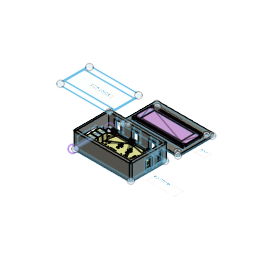
FurModularity case (Autodesk Fusion 360 design; units mm, degrees)
part number: 2026-01-23-19-48-48-350
Autodesk Fusion 360 part; units mm, degrees
sketch "Esboço1" plane through (0, 0, 0) normal (0, 1, 0) x (1, 0, 0)
  line L0 (-156.1961, 83) -> (-258.1961, 83)
  line L1 (-258.1961, 83) -> (-258.1961, 23)
  line L2 (-258.1961, 23) -> (-156.1961, 23)
  line L3 (-156.1961, 23) -> (-156.1961, 83)
  line L4 (-261.1961, 88) -> (-151.1961, 88)
  line L5 (-151.1961, 88) -> (-151.1961, 18)
  line L6 (-151.1961, 18) -> (-261.1961, 18)
  line L7 (-261.1961, 18) -> (-261.1961, 88)
  circle A0 centre (-258.6961, 20.5) radius 1.7
  circle A1 centre (-153.6961, 20.5) radius 1.7
  circle A2 centre (-153.6961, 85.5) radius 1.7
  circle A3 centre (-258.6961, 85.5) radius 1.7
  line L8 (-382.0556, 170.4962) -> (-284.0556, 170.4962)
  line L9 (-284.0556, 170.4962) -> (-284.0556, 110.4962)
  line L10 (-284.0556, 110.4962) -> (-382.0556, 110.4962)
  line L11 (-382.0556, 110.4962) -> (-382.0556, 170.4962)
  circle A4 centre (-379.5556, 167.9962) radius 1.25
  circle A5 centre (-379.5556, 112.9962) radius 1.25
  circle A6 centre (-286.5556, 112.9962) radius 1.25
  circle A7 centre (-286.5556, 167.9962) radius 1.25
  line L12 (-380.2556, 159.1962) -> (-285.8556, 159.1962)
  line L13 (-285.8556, 159.1962) -> (-285.8556, 121.7962)
  line L14 (-285.8556, 121.7962) -> (-380.2556, 121.7962)
  line L15 (-380.2556, 121.7962) -> (-380.2556, 159.1962)
  line L16 (-148.0106, 174.0206) -> (-148.0106, 104.0206)
  line L17 (-148.0106, 104.0206) -> (-258.0106, 104.0206)
  line L18 (-258.0106, 104.0206) -> (-258.0106, 174.0206)
  line L19 (-258.0106, 174.0206) -> (-148.0106, 174.0206)
  circle A8 centre (-255.5106, 171.5206) radius 1.5
  circle A9 centre (-150.5106, 171.5206) radius 1.5
  circle A10 centre (-255.5106, 106.5206) radius 1.5
  circle A11 centre (-150.5106, 106.5206) radius 1.5
  line L20 (-348.3038, 137.4104) -> (-309.3267, 137.4104) construction
  line L21 (-309.3267, 137.4104) -> (-309.3267, 143.3671) construction
  line L22 (-309.3267, 143.3671) -> (-348.3038, 143.3671) construction
  line L23 (-348.3038, 143.3671) -> (-348.3038, 137.4104) construction
  line L24 (-139.2514, 36.3126) -> (-87.0034, 36.3126) construction
  line L25 (-87.0034, 36.3126) -> (-87.0034, 53) construction
  line L26 (-87.0034, 53) -> (-139.2514, 53) construction
  line L27 (-139.2514, 53) -> (-139.2514, 36.3126) construction
  circle A12 centre (-249.5106, 111.5206) radius 1.25
  line L28 (-155.8106, 120.3206) -> (-250.2106, 120.3206)
  line L29 (-250.2106, 157.7206) -> (-155.8106, 157.7206)
  line L30 (-250.2106, 120.3206) -> (-250.2106, 157.7206)
  circle A13 centre (-156.5106, 166.5206) radius 1.25
  circle A14 centre (-249.5106, 166.5206) radius 1.25
  circle A15 centre (-156.5106, 111.5206) radius 1.25
  line L31 (-155.8106, 157.7206) -> (-155.8106, 120.3206)
  line L32 (-140, 128.1599) -> (-121.0217, 128.1599) construction
  line L33 (-121.0217, 128.1599) -> (-121.0217, 140) construction
  line L34 (-121.0217, 140) -> (-140, 140) construction
  line L35 (-140, 140) -> (-140, 128.1599) construction
  dimension "d17" = 60
  dimension "d18" = 102
  dimension "d19" = 110
  dimension "d20" = 70
  dimension "d22" = 5
  dimension "d25" = 3.4
  dimension "d27" = 2.5
  dimension "d28" = 2.5
  dimension "d29" = 3.4
  dimension "d30" = 2.5
  dimension "d31" = 2.5
  dimension "d32" = 3.4
  dimension "d33" = 3.4
  dimension "d34" = 2.5
  dimension "d35" = 2.5
  dimension "d36" = 2.5
  dimension "d37" = 2.5
  dimension "d54" = 60
  dimension "d55" = 98
  dimension "d60" = 2.5
  dimension "d61" = 2.5
  dimension "d62" = 2.5
  dimension "d63" = 2.5
  dimension "d64" = 2.5
  dimension "d65" = 2.5
  dimension "d66" = 2.5
  dimension "d67" = 2.5
  dimension "d68" = 2.5
  dimension "d69" = 2.5
  dimension "d70" = 2.5
  dimension "d71" = 2.5
  dimension "d73" = 94.4
  dimension "d74" = 37.4
  dimension "d75" = 1.8
  dimension "d76" = 11.3
  dimension "d77" = 70
  dimension "d78" = 110
  dimension "d79" = 3
  dimension "d80" = 3
  dimension "d82" = 3
  dimension "d83" = 2.5
  dimension "d85" = 2.5
  dimension "d86" = 2.5
  dimension "d87" = 2.5
  dimension "d88" = 3
  dimension "d89" = 2.5
  dimension "d90" = 2.5
  dimension "d91" = 2.5
  dimension "d92" = 2.5
  dimension "d93" = 5
  dimension "d94" = 0
  dimension "d95" = 5
  dimension "d105" = 2.5
  dimension "d108" = 2.5
  dimension "d111" = 2.5
  dimension "d114" = 2.5
  dimension "d117" = 94.4
  dimension "d118" = 37.4
  dimension "d121" = 93
  dimension "d122" = 55
  dimension "d124" = 93
  dimension "d125" = 8.8
  dimension "d126" = 8.8
  dimension "d127" = 0.7
  dimension "d129" = 7.5
  dimension "d132" = 5
  dimension "d135" = 8.5
  dimension "d173" = 5
  constraint horizontal L0
  constraint vertical L1
  constraint horizontal L2
  constraint vertical L3
  constraint horizontal L4
  constraint vertical L5
  constraint horizontal L6
  constraint vertical L7
  constraint horizontal L8
  constraint vertical L9
  constraint horizontal L10
  constraint vertical L11
  constraint horizontal L12
  constraint vertical L13
  constraint horizontal L14
  constraint vertical L15
  constraint vertical L16
  constraint horizontal L17
  constraint vertical L18
  constraint perpendicular L16 L19
  constraint horizontal L29
  constraint vertical L31
  constraint horizontal L28
  constraint vertical L30
  measures "d17" distance of L0.start L2.end
  measures "d18" distance of L0.start L0.end
  measures "d19" distance of L4.start L4.end
  measures "d20" distance of L4.start L6.end
  measures "d22" distance of L0 L4
  measures "d25" diameter of A0
  measures "d27" distance of L7 A0.centre
  measures "d28" distance of L6 A0.centre
  measures "d29" diameter of A1
  measures "d30" distance of L5 A1.centre
  measures "d31" distance of L6 A1.centre
  measures "d32" diameter of A3
  measures "d33" diameter of A2
  measures "d34" distance of L4 A2.centre
  measures "d35" distance of L5 A2.centre
  measures "d36" distance of L4 A3.centre
  measures "d37" distance of L7 A3.centre
  measures "d54" distance of L8.start L10.end
  measures "d55" distance of L8.start L8.end
  measures "d60" diameter of A4
  measures "d61" distance of L8 A4.centre
  measures "d62" distance of L11 A4.centre
  measures "d63" diameter of A5
  measures "d64" distance of L10 A5.centre
  measures "d65" distance of L11 A5.centre
  measures "d66" diameter of A6
  measures "d67" distance of L9 A6.centre
  measures "d68" distance of L10 A6.centre
  measures "d69" diameter of A7
  measures "d70" distance of L8 A7.centre
  measures "d71" distance of L9 A7.centre
  measures "d73" distance of L12.start L12.end
  measures "d74" distance of L12.start L14.end
  measures "d75" distance of L11 L15
  measures "d76" distance of L10 L14
  measures "d77" distance of L18.end L17.end
  measures "d78" distance of L18.end L16.start
  measures "d79" diameter of A8
  measures "d80" diameter of A9
  measures "d82" diameter of A10
  measures "d83" distance of L19 A8.centre
  measures "d85" distance of L18 A8.centre
  measures "d86" distance of L19 A9.centre
  measures "d87" distance of L16 A9.centre
  measures "d88" diameter of A11
  measures "d89" distance of L16 A11.centre
  measures "d90" distance of L17 A11.centre
  measures "d91" distance of L17 A10.centre
  measures "d92" distance of L18 A10.centre
  measures "d105" diameter of A14
  measures "d108" diameter of A12
  measures "d111" diameter of A15
  measures "d114" diameter of A13
  measures "d117" distance of L29.start L29.end
  measures "d118" distance of L29.start L28.end
  measures "d121" distance of A15.centre A12.centre
  measures "d122" distance of A14.centre A12.centre
  measures "d124" distance of A14.centre A13.centre
  measures "d125" distance of A14.centre L29
  measures "d126" distance of A15.centre L28
  measures "d127" distance of A14.centre L30
  measures "d129" distance of L19 A14.centre
  measures "d135" distance of L18 A14.centre
  measures "d173" distance of L3 L5
other "Recurso de malha base1"
other "Modificar1"
other "Modificar2"
other "Modificar3"
other "Modificar4"
other "Recurso de malha base2"
other "Modificar5"
other "Modificar6"
other "Modificar7"
other "Modificar8"
extrude "Extrusão18" add sketch "Esboço1" along normal blind 30 contours L4 L5 L6 L7 makes body 1
extrude "Extrusão19" add sketch "Esboço1" along normal blind 3 separate body contours L0 L1 L2 L3 | A0 | A1 | A2 | A3 makes body 2 at (-258.2357, 2, -87.1365) makes body 3 at (-153.6537, 2, -87.1995) makes body 4 at (-258.2357, 2, -22.1365) makes body 5 at (-190.1961, 0, -63) makes body 6 at (-153.6537, 2, -22.1995)
sketch "Esboço4" plane through (-261.1961, 0, 0) normal (-1, 0, 0) x (0, 0, 1)
  line L0 (-88, 0) -> (-18, 0)
  line L1 (-18, 0) -> (-18, 30)
  line L2 (-18, 30) -> (-88, 30)
  line L3 (-88, 30) -> (-88, 0)
  line L4 (-18, 0) -> (-88, 0)
  line L5 (-73.7635, 9.0114) -> (-62.7635, 9.0114)
  line L6 (-62.7635, 9.0114) -> (-62.7635, 2.0114)
  line L7 (-62.7635, 2.0114) -> (-73.7635, 2.0114)
  line L8 (-73.7635, 2.0114) -> (-73.7635, 9.0114)
  line L9 (-61.7, 16.0562) -> (-27.0978, 16.0562)
  line L10 (-27.0978, 16.0562) -> (-27.0978, 3.9829)
  line L11 (-27.0978, 3.9829) -> (-61.7, 3.9829)
  line L12 (-61.7, 3.9829) -> (-61.7, 16.0562)
  point P0 (-58.6316, 10.8)
  dimension "d184" = 7
  dimension "d185" = 11
  constraint horizontal L5
  constraint vertical L6
  constraint horizontal L7
  constraint vertical L8
  constraint horizontal L9
  constraint vertical L10
  constraint horizontal L11
  constraint vertical L12
  measures "d184" distance of L5 L7
  measures "d185" distance of L6 L8
extrude "Extrusão20" cut sketch "Esboço4" against normal blind 3 contours L5 L6 L7 L8 | L9 L10 L11 L12 bodies 1
extrude "Extrusão21" add sketch "Esboço1" along normal blind 3 separate body contours L16 L17 L18 L19 makes body 7
sketch "Esboço5" plane through (0, 0, -88) normal (0, 0, -1) x (-1, 0, 0)
  line L0 (151.1961, 0) -> (261.1961, 0)
  line L1 (261.1961, 0) -> (261.1961, 30)
  line L2 (261.1961, 30) -> (151.1961, 30)
  line L3 (151.1961, 30) -> (151.1961, 0)
  line L4 (170.1901, 3.9119) -> (182.6901, 3.9119)
  line L5 (182.6901, 3.9119) -> (182.6901, 23.4119)
  line L6 (182.6901, 23.4119) -> (170.1901, 23.4119)
  line L7 (170.1901, 23.4119) -> (170.1901, 3.9119)
  line L8 (202.5128, 23.2516) -> (215.0128, 23.2516)
  line L9 (215.0128, 23.2516) -> (215.0128, 3.7516)
  line L10 (215.0128, 3.7516) -> (202.5128, 3.7516)
  line L11 (202.5128, 3.7516) -> (202.5128, 23.2516)
  line L12 (235.1378, 23.3674) -> (247.6378, 23.3674)
  line L13 (247.6378, 23.3674) -> (247.6378, 3.8674)
  line L14 (247.6378, 3.8674) -> (235.1378, 3.8674)
  line L15 (235.1378, 3.8674) -> (235.1378, 23.3674)
  dimension "d190" = 12.5
  dimension "d191" = 19.5
  dimension "d192" = 12.5
  dimension "d193" = 19.5
  dimension "d194" = 12.5
  dimension "d195" = 19.5
  constraint horizontal L4
  constraint vertical L5
  constraint horizontal L6
  constraint vertical L7
  constraint horizontal L8
  constraint vertical L9
  constraint horizontal L10
  constraint vertical L11
  constraint horizontal L12
  constraint vertical L13
  constraint horizontal L14
  constraint vertical L15
  measures "d190" distance of L5 L7
  measures "d191" distance of L4 L6
  measures "d192" distance of L8.start L8.end
  measures "d193" distance of L8.start L10.end
  measures "d194" distance of L12.start L12.end
  measures "d195" distance of L12.start L14.end
extrude "Extrusão22" cut sketch "Esboço5" against normal blind 5 contours L4 L5 L6 L7 | L8 L9 L10 L11 bodies 1
sketch "Esboço6" plane through (-151.1961, 0, 0) normal (1, 0, 0) x (0, 0, -1)
  line L0 (18, 0) -> (88, 0)
  line L1 (88, 0) -> (88, 30)
  line L2 (88, 30) -> (18, 30)
  line L3 (18, 30) -> (18, 0)
  line L4 (66.1419, 23.3852) -> (78.6419, 23.3852)
  line L5 (78.6419, 23.3852) -> (78.6419, 3.8852)
  line L6 (78.6419, 3.8852) -> (66.1419, 3.8852)
  line L7 (66.1419, 3.8852) -> (66.1419, 23.3852)
  line L8 (46.1614, 23.386) -> (58.6614, 23.386)
  line L9 (58.6614, 23.386) -> (58.6614, 3.886)
  line L10 (58.6614, 3.886) -> (46.1614, 3.886)
  line L11 (46.1614, 3.886) -> (46.1614, 23.386)
  dimension "d198" = 12.5
  dimension "d199" = 19.5
  dimension "d200" = 12.5
  dimension "d201" = 19.5
  constraint horizontal L4
  constraint vertical L5
  constraint horizontal L6
  constraint vertical L7
  constraint horizontal L8
  constraint vertical L9
  constraint horizontal L10
  constraint vertical L11
  measures "d198" distance of L4.start L4.end
  measures "d199" distance of L4.start L6.end
  measures "d200" distance of L8.start L8.end
  measures "d201" distance of L8.start L10.end
extrude "Extrusão23" cut sketch "Esboço6" against normal blind 5 contours L4 L5 L6 L7 | L8 L9 L10 L11 bodies 1
extrude "Extrusão24" cut sketch "Esboço6" against normal blind 5 contours L4 L5 L6 L7 | L8 L9 L10 L11 bodies 1
extrude "Extrusão25" cut sketch "Esboço5" against normal blind 5 contours L12 L13 L14 L15 bodies 1
fillet "Arredondamento3" radius 2.5 4 edges at (-261.1961, 15, -88) (-261.1961, 15, -18) (-151.1961, 15, -18) (-151.1961, 15, -88) on bodies 1
fillet "Arredondamento4" radius 2.5 4 edges at (-148.0106, 1.5, -174.0206) (-258.0106, 1.5, -174.0206) (-258.0106, 1.5, -104.0206) (-148.0106, 1.5, -104.0206) on bodies 7
extrude "Extrusão9" [suppressed]
extrude "Extrusão10" [suppressed]
extrude "Extrusão7" [suppressed]
extrude "Extrusão8" [suppressed]
equation "d94 = 'LCD 20x04'"
equation "d96 = 'BOTTOM'"
equation "d133 = 'TOP'"
